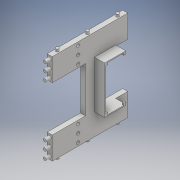
# Autodesk Inventor part: Side Panels V2
Saved by Autodesk Inventor 2017.3 (Build 213256000, 256)
## iProperties
Created: 2018-03-06
Part Number: Side Panels V2
Material: Generic
Document SubType Name: Modeling
Designer: Harsh Gupta
Density: 1 g/cm^3
Appearance: Default
Author: Harsh Gupta
Autodesk Inventor part; units mm, degrees
ref_plane "YZ Plane" through (0, 0, 0) normal (1, 0, 0) x (0, 1, 0)
sketch "Sketch1" plane through (0, 0, 0) normal (0, 1, 0) x (-1, 0, 0)
  line L0 (0, 0) -> (5, 0)
  line L1 (5, 0) -> (5, -90)
  line L2 (5, -90) -> (0, -90)
  line L3 (0, -90) -> (0, 0)
  dimension "d0" = 5
  dimension "d1" = 90
  constraints: 8 end point, 2 parallel, 1 horizontal, 1 perpendicular
  measures "d0" distance of L1.end L2.end
  measures "d1" distance of L0.end L1.end
extrude "Extrusion1" add sketch "Sketch1" along normal blind 75
sketch "Sketch2" plane through (0, 0, 0) normal (1, 0, 0) x (0, 0, -1)
  line L0 (90, 0) -> (0, 0) projected
  line L1 (22.5, 0) -> (67.5, 0)
  line L2 (67.5, 0) -> (67.5, 33)
  line L3 (67.5, 33) -> (22.5, 33)
  line L4 (22.5, 33) -> (22.5, 0)
  line L5 (0, 0) -> (0, 75) projected
  line L6 (90, 0) -> (90, 75) projected
  line L7 (22.5, 43) -> (67.5, 43)
  line L8 (67.5, 43) -> (67.5, 75)
  line L9 (67.5, 75) -> (22.5, 75)
  line L10 (22.5, 75) -> (22.5, 43)
  line L11 (0, 75) -> (90, 75) projected
  dimension "d4" = 45
  dimension "d5" = 22.5
  dimension "d6" = 22.5
  dimension "d7" = 33
  dimension "d8" = 10
  dimension "d9" = 22.5
  dimension "d10" = 22.5
  constraints: 16 end point, 4 parallel, 2 horizontal, 2 perpendicular, 1 collinear, 1 point on line
  measures "d4" distance of L3.end L2.end
  measures "d5" distance between parallel lines of L5 L4
  measures "d6" distance between parallel lines of L6 L2
  measures "d7" distance of L3.end L1.start
  measures "d8" distance between parallel lines of L7 L3
  measures "d9" distance between parallel lines of L5 L10
  measures "d10" distance between parallel lines of L6 L8
extrude "Extrusion2" cut sketch "Sketch2" against normal through all contours L0 L4 L3 L2 | L8 L7 L10 L9
sketch "Sketch3" plane through (0, 0, 0) normal (1, 0, 0) x (0, 0, -1)
  line L0 (67.5, 43) -> (22.5, 43) projected
  line L1 (67.5, 63) -> (67.5, 43) projected
  line L2 (22.5, 63) -> (67.5, 63) projected
  line L3 (22.5, 43) -> (22.5, 63) projected
  circle A0 centre (23.5, 44) radius 0.75 projected
  circle A1 centre (23.5, 62) radius 0.75 projected
  circle A2 centre (66.5, 44) radius 0.75 projected
  circle A3 centre (66.5, 62) radius 0.75 projected
  line L4 (42.55, 45.5) -> (42.35, 45.5) projected
  line L5 (42.55, 45.5) -> (42.65, 45.6) projected
  line L6 (44.8, 45.6) -> (42.65, 45.6) projected
  line L7 (44.8, 45.6) -> (44.9, 45.5) projected
  line L8 (45.1, 45.5) -> (44.9, 45.5) projected
  line L9 (45.1, 45.5) -> (45.2, 45.6) projected
  line L10 (47.35, 45.6) -> (45.2, 45.6) projected
  line L11 (47.35, 45.6) -> (47.45, 45.5) projected
  line L12 (47.65, 45.5) -> (47.45, 45.5) projected
  line L13 (47.65, 45.5) -> (47.75, 45.6) projected
  line L14 (49.9, 45.6) -> (47.75, 45.6) projected
  line L15 (49.9, 45.6) -> (50, 45.5) projected
  line L16 (50, 43.2) -> (50, 45.5) projected
  line L17 (50, 43.2) -> (49.9, 43.1) projected
  line L18 (47.75, 43.1) -> (49.9, 43.1) projected
  line L19 (47.75, 43.1) -> (47.65, 43.2) projected
  line L20 (47.45, 43.2) -> (47.65, 43.2) projected
  line L21 (47.45, 43.2) -> (47.35, 43.1) projected
  line L22 (45.2, 43.1) -> (47.35, 43.1) projected
  line L23 (45.2, 43.1) -> (45.1, 43.2) projected
  line L24 (44.9, 43.2) -> (45.1, 43.2) projected
  line L25 (44.9, 43.2) -> (44.8, 43.1) projected
  line L26 (42.65, 43.1) -> (44.8, 43.1) projected
  line L27 (42.65, 43.1) -> (42.55, 43.2) projected
  line L28 (42.35, 43.2) -> (42.55, 43.2) projected
  line L29 (42.35, 43.2) -> (42.25, 43.1) projected
  line L30 (40.1, 43.1) -> (42.25, 43.1) projected
  line L31 (40.1, 43.1) -> (40, 43.2) projected
  line L32 (40, 45.5) -> (40, 43.2) projected
  line L33 (40, 45.5) -> (40.1, 45.6) projected
  line L34 (42.25, 45.6) -> (40.1, 45.6) projected
  line L35 (42.25, 45.6) -> (42.35, 45.5) projected
  line L36 (24, 56.95) -> (24, 56.75) projected
  line L37 (24.1, 56.95) -> (24, 56.95) projected
  line L38 (24.1, 56.75) -> (24.1, 56.95) projected
  line L39 (24, 56.75) -> (24.1, 56.75) projected
  line L40 (28.9, 56.95) -> (28.9, 56.75) projected
  line L41 (29, 56.95) -> (28.9, 56.95) projected
  line L42 (29, 56.75) -> (29, 56.95) projected
  line L43 (28.9, 56.75) -> (29, 56.75) projected
  line L44 (24, 55.8071) -> (24, 55.6071) projected
  line L45 (24.1, 55.8071) -> (24, 55.8071) projected
  line L46 (24.1, 55.6071) -> (24.1, 55.8071) projected
  line L47 (24, 55.6071) -> (24.1, 55.6071) projected
  line L48 (28.9, 55.8071) -> (28.9, 55.6071) projected
  line L49 (29, 55.8071) -> (28.9, 55.8071) projected
  line L50 (29, 55.6071) -> (29, 55.8071) projected
  line L51 (28.9, 55.6071) -> (29, 55.6071) projected
  line L52 (24, 54.6643) -> (24, 54.4643) projected
  line L53 (24.1, 54.6643) -> (24, 54.6643) projected
  line L54 (24.1, 54.4643) -> (24.1, 54.6643) projected
  line L55 (24, 54.4643) -> (24.1, 54.4643) projected
  line L56 (28.9, 54.6643) -> (28.9, 54.4643) projected
  line L57 (29, 54.6643) -> (28.9, 54.6643) projected
  line L58 (29, 54.4643) -> (29, 54.6643) projected
  line L59 (28.9, 54.4643) -> (29, 54.4643) projected
  line L60 (24, 53.5214) -> (24, 53.3214) projected
  line L61 (24.1, 53.5214) -> (24, 53.5214) projected
  line L62 (24.1, 53.3214) -> (24.1, 53.5214) projected
  line L63 (24, 53.3214) -> (24.1, 53.3214) projected
  line L64 (28.9, 53.5214) -> (28.9, 53.3214) projected
  line L65 (29, 53.5214) -> (28.9, 53.5214) projected
  line L66 (29, 53.3214) -> (29, 53.5214) projected
  line L67 (28.9, 53.3214) -> (29, 53.3214) projected
  line L68 (24, 52.3786) -> (24, 52.1786) projected
  line L69 (24.1, 52.3786) -> (24, 52.3786) projected
  line L70 (24.1, 52.1786) -> (24.1, 52.3786) projected
  line L71 (24, 52.1786) -> (24.1, 52.1786) projected
  line L72 (28.9, 52.3786) -> (28.9, 52.1786) projected
  line L73 (29, 52.3786) -> (28.9, 52.3786) projected
  line L74 (29, 52.1786) -> (29, 52.3786) projected
  line L75 (28.9, 52.1786) -> (29, 52.1786) projected
  line L76 (24, 51.2357) -> (24, 51.0357) projected
  line L77 (24.1, 51.2357) -> (24, 51.2357) projected
  line L78 (24.1, 51.0357) -> (24.1, 51.2357) projected
  line L79 (24, 51.0357) -> (24.1, 51.0357) projected
  line L80 (28.9, 51.2357) -> (28.9, 51.0357) projected
  line L81 (29, 51.2357) -> (28.9, 51.2357) projected
  line L82 (29, 51.0357) -> (29, 51.2357) projected
  line L83 (28.9, 51.0357) -> (29, 51.0357) projected
  line L84 (24, 50.0929) -> (24, 49.8929) projected
  line L85 (24.1, 50.0929) -> (24, 50.0929) projected
  line L86 (24.1, 49.8929) -> (24.1, 50.0929) projected
  line L87 (24, 49.8929) -> (24.1, 49.8929) projected
  line L88 (28.9, 50.0929) -> (28.9, 49.8929) projected
  line L89 (29, 50.0929) -> (28.9, 50.0929) projected
  line L90 (29, 49.8929) -> (29, 50.0929) projected
  line L91 (28.9, 49.8929) -> (29, 49.8929) projected
  line L92 (24, 48.95) -> (24, 48.75) projected
  line L93 (24.1, 48.95) -> (24, 48.95) projected
  line L94 (24.1, 48.75) -> (24.1, 48.95) projected
  line L95 (24, 48.75) -> (24.1, 48.75) projected
  line L96 (28.9, 48.95) -> (28.9, 48.75) projected
  line L97 (29, 48.95) -> (28.9, 48.95) projected
  line L98 (29, 48.75) -> (29, 48.95) projected
  line L99 (28.9, 48.75) -> (29, 48.75) projected
  line L100 (40.95, 50.5) -> (41.15, 50.5) projected
  line L101 (40.95, 50.55) -> (40.95, 50.5) projected
  line L102 (41.15, 50.55) -> (40.95, 50.55) projected
  line L103 (41.15, 50.5) -> (41.15, 50.55) projected
  line L104 (41.15, 55.5) -> (40.95, 55.5) projected
  line L105 (41.15, 55.45) -> (41.15, 55.5) projected
  line L106 (40.95, 55.45) -> (41.15, 55.45) projected
  line L107 (40.95, 55.5) -> (40.95, 55.45) projected
  line L108 (42.2667, 50.5) -> (42.4667, 50.5) projected
  line L109 (42.2667, 50.55) -> (42.2667, 50.5) projected
  line L110 (42.4667, 50.55) -> (42.2667, 50.55) projected
  line L111 (42.4667, 50.5) -> (42.4667, 50.55) projected
  line L112 (42.4667, 55.5) -> (42.2667, 55.5) projected
  line L113 (42.4667, 55.45) -> (42.4667, 55.5) projected
  line L114 (42.2667, 55.45) -> (42.4667, 55.45) projected
  line L115 (42.2667, 55.5) -> (42.2667, 55.45) projected
  line L116 (43.5833, 50.5) -> (43.7833, 50.5) projected
  line L117 (43.5833, 50.55) -> (43.5833, 50.5) projected
  line L118 (43.7833, 50.55) -> (43.5833, 50.55) projected
  line L119 (43.7833, 50.5) -> (43.7833, 50.55) projected
  line L120 (43.7833, 55.5) -> (43.5833, 55.5) projected
  line L121 (43.7833, 55.45) -> (43.7833, 55.5) projected
  line L122 (43.5833, 55.45) -> (43.7833, 55.45) projected
  line L123 (43.5833, 55.5) -> (43.5833, 55.45) projected
  line L124 (44.9, 50.5) -> (45.1, 50.5) projected
  line L125 (44.9, 50.55) -> (44.9, 50.5) projected
  line L126 (45.1, 50.55) -> (44.9, 50.55) projected
  line L127 (45.1, 50.5) -> (45.1, 50.55) projected
  line L128 (45.1, 55.5) -> (44.9, 55.5) projected
  line L129 (45.1, 55.45) -> (45.1, 55.5) projected
  line L130 (44.9, 55.45) -> (45.1, 55.45) projected
  line L131 (44.9, 55.5) -> (44.9, 55.45) projected
  line L132 (46.2167, 50.5) -> (46.4167, 50.5) projected
  line L133 (46.2167, 50.55) -> (46.2167, 50.5) projected
  line L134 (46.4167, 50.55) -> (46.2167, 50.55) projected
  line L135 (46.4167, 50.5) -> (46.4167, 50.55) projected
  line L136 (46.4167, 55.5) -> (46.2167, 55.5) projected
  line L137 (46.4167, 55.45) -> (46.4167, 55.5) projected
  line L138 (46.2167, 55.45) -> (46.4167, 55.45) projected
  line L139 (46.2167, 55.5) -> (46.2167, 55.45) projected
  line L140 (47.5333, 50.5) -> (47.7333, 50.5) projected
  line L141 (47.5333, 50.55) -> (47.5333, 50.5) projected
  line L142 (47.7333, 50.55) -> (47.5333, 50.55) projected
  line L143 (47.7333, 50.5) -> (47.7333, 50.55) projected
  line L144 (47.7333, 55.5) -> (47.5333, 55.5) projected
  line L145 (47.7333, 55.45) -> (47.7333, 55.5) projected
  line L146 (47.5333, 55.45) -> (47.7333, 55.45) projected
  line L147 (47.5333, 55.5) -> (47.5333, 55.45) projected
  line L148 (48.85, 50.5) -> (49.05, 50.5) projected
  line L149 (48.85, 50.55) -> (48.85, 50.5) projected
  line L150 (49.05, 50.55) -> (48.85, 50.55) projected
  line L151 (49.05, 50.5) -> (49.05, 50.55) projected
  line L152 (49.05, 55.5) -> (48.85, 55.5) projected
  line L153 (49.05, 55.45) -> (49.05, 55.5) projected
  line L154 (48.85, 55.45) -> (49.05, 55.45) projected
  line L155 (48.85, 55.5) -> (48.85, 55.45) projected
  line L156 (59.1, 50.5) -> (59.3, 50.5) projected
  line L157 (59.1, 50.55) -> (59.1, 50.5) projected
  line L158 (59.3, 50.55) -> (59.1, 50.55) projected
  line L159 (59.3, 50.5) -> (59.3, 50.55) projected
  line L160 (59.3, 55.5) -> (59.1, 55.5) projected
  line L161 (59.3, 55.45) -> (59.3, 55.5) projected
  line L162 (59.1, 55.45) -> (59.3, 55.45) projected
  line L163 (59.1, 55.5) -> (59.1, 55.45) projected
  line L164 (60.4167, 50.5) -> (60.6167, 50.5) projected
  line L165 (60.4167, 50.55) -> (60.4167, 50.5) projected
  line L166 (60.6167, 50.55) -> (60.4167, 50.55) projected
  line L167 (60.6167, 50.5) -> (60.6167, 50.55) projected
  line L168 (60.6167, 55.5) -> (60.4167, 55.5) projected
  line L169 (60.6167, 55.45) -> (60.6167, 55.5) projected
  line L170 (60.4167, 55.45) -> (60.6167, 55.45) projected
  line L171 (60.4167, 55.5) -> (60.4167, 55.45) projected
  line L172 (61.7333, 50.5) -> (61.9333, 50.5) projected
  line L173 (61.7333, 50.55) -> (61.7333, 50.5) projected
  line L174 (61.9333, 50.55) -> (61.7333, 50.55) projected
  line L175 (61.9333, 50.5) -> (61.9333, 50.55) projected
  line L176 (61.9333, 55.5) -> (61.7333, 55.5) projected
  line L177 (61.9333, 55.45) -> (61.9333, 55.5) projected
  line L178 (61.7333, 55.45) -> (61.9333, 55.45) projected
  line L179 (61.7333, 55.5) -> (61.7333, 55.45) projected
  line L180 (63.05, 50.5) -> (63.25, 50.5) projected
  line L181 (63.05, 50.55) -> (63.05, 50.5) projected
  line L182 (63.25, 50.55) -> (63.05, 50.55) projected
  line L183 (63.25, 50.5) -> (63.25, 50.55) projected
  line L184 (63.25, 55.5) -> (63.05, 55.5) projected
  line L185 (63.25, 55.45) -> (63.25, 55.5) projected
  line L186 (63.05, 55.45) -> (63.25, 55.45) projected
  line L187 (63.05, 55.5) -> (63.05, 55.45) projected
  line L188 (64.3667, 50.5) -> (64.5667, 50.5) projected
  line L189 (64.3667, 50.55) -> (64.3667, 50.5) projected
  line L190 (64.5667, 50.55) -> (64.3667, 50.55) projected
  line L191 (64.5667, 50.5) -> (64.5667, 50.55) projected
  line L192 (64.5667, 55.5) -> (64.3667, 55.5) projected
  line L193 (64.5667, 55.45) -> (64.5667, 55.5) projected
  line L194 (64.3667, 55.45) -> (64.5667, 55.45) projected
  line L195 (64.3667, 55.5) -> (64.3667, 55.45) projected
  line L196 (65.6833, 50.5) -> (65.8833, 50.5) projected
  line L197 (65.6833, 50.55) -> (65.6833, 50.5) projected
  line L198 (65.8833, 50.55) -> (65.6833, 50.55) projected
  line L199 (65.8833, 50.5) -> (65.8833, 50.55) projected
  line L200 (65.8833, 55.5) -> (65.6833, 55.5) projected
  line L201 (65.8833, 55.45) -> (65.8833, 55.5) projected
  line L202 (65.6833, 55.45) -> (65.8833, 55.45) projected
  line L203 (65.6833, 55.5) -> (65.6833, 55.45) projected
  line L204 (67, 50.5) -> (67.2, 50.5) projected
  line L205 (67, 50.55) -> (67, 50.5) projected
  line L206 (67.2, 50.55) -> (67, 50.55) projected
  line L207 (67.2, 50.5) -> (67.2, 50.55) projected
  line L208 (67.2, 55.5) -> (67, 55.5) projected
  line L209 (67.2, 55.45) -> (67.2, 55.5) projected
  line L210 (67, 55.45) -> (67.2, 55.45) projected
  line L211 (67, 55.5) -> (67, 55.45) projected
  line L212 (58.9, 55) -> (58.9, 51) projected
  line L213 (67.4, 55) -> (58.9, 55) projected
  line L214 (67.4, 51) -> (67.4, 55) projected
  line L215 (58.9, 51) -> (67.4, 51) projected
  line L216 (49.25, 51) -> (49.25, 55) projected
  line L217 (40.75, 51) -> (49.25, 51) projected
  line L218 (40.75, 55) -> (40.75, 51) projected
  line L219 (49.25, 55) -> (40.75, 55) projected
  line L220 (24.5, 57.75) -> (24.5, 48.25) projected
  line L221 (28.5, 57.75) -> (24.5, 57.75) projected
  line L222 (28.5, 48.25) -> (28.5, 57.75) projected
  line L223 (24.5, 48.25) -> (28.5, 48.25) projected
  line L224 (22.5, 63) -> (21.5, 63)
  line L225 (21.5, 63) -> (21.5, 42)
  line L226 (21.5, 42) -> (22.5, 42)
  line L227 (22.5, 43) -> (22.5, 63)
  line L228 (67.5, 63) -> (68.5, 63)
  line L229 (68.5, 63) -> (68.5, 42)
  line L230 (68.5, 42) -> (67.5, 42)
  line L231 (67.5, 43) -> (67.5, 63)
  line L232 (67.5, 75) -> (67.5, 43) projected
  line L233 (22.5, 42) -> (67.5, 42)
  line L234 (67.5, 43) -> (22.5, 43)
  point P0 (0, 0)
  dimension "d13" = 1
  dimension "d14" = 21
  dimension "d15" = 1
  dimension "d17" = 47
  constraints: 20 end point, 5 parallel, 3 horizontal, 2 perpendicular, 2 point on line, 1 collinear
  measures "d13" distance of L226.end L225.end
  measures "d14" distance of L225.end L224.end
  measures "d15" distance of L229.end L230.end
  measures "d17" distance of L225.end L229.end
extrude "Extrusion3" add sketch "Sketch3" along normal blind 10 contours L1 L228 L229 L230 L233 L226 L225 L224 L3 L0
ref_plane "Work Plane1" through (8.43, 53, 385.6573) normal (1, 0, 0) x (0, 0, -1)
sketch "Sketch4" plane through (8.43, 53, 385.6573) normal (1, 0, 0) x (0, 0, -1)
  line L0 (408.1573, -10) -> (408.1573, 10) projected
  line L1 (408.1573, 10) -> (410.1573, 10)
  line L2 (410.1573, 10) -> (410.1573, 8)
  line L3 (410.1573, 8) -> (408.1573, 8)
  line L4 (408.1573, 8) -> (408.1573, 10)
  line L5 (453.1573, -10) -> (408.1573, -10) projected
  line L6 (408.1573, -10) -> (410.1573, -10)
  line L7 (410.1573, -10) -> (410.1573, -8)
  line L8 (410.1573, -8) -> (408.1573, -8)
  line L9 (408.1573, -8) -> (408.1573, -10)
  line L10 (234.5466, 10) -> (234.5466, -10) projected
  line L11 (453.1573, -10) -> (451.1573, -10)
  line L12 (451.1573, -10) -> (451.1573, -8)
  line L13 (451.1573, -8) -> (453.1573, -8)
  line L14 (453.1573, -8) -> (453.1573, -10)
  line L15 (453.1573, 10) -> (451.1573, 10)
  line L16 (451.1573, 10) -> (451.1573, 8)
  line L17 (451.1573, 8) -> (453.1573, 8)
  line L18 (453.1573, 8) -> (453.1573, 10)
  point P0 (385.6573, -53)
  dimension "d20" = 2
  dimension "d21" = 2
  dimension "d22" = 2
  dimension "d23" = 2
  dimension "d24" = 2
  dimension "d25" = 2
  dimension "d26" = 2
  dimension "d27" = 2
  constraints: 32 end point, 8 parallel, 4 horizontal, 4 perpendicular
  measures "d20" distance of L2.end L3.end
  measures "d21" distance of L1.end L2.end
  measures "d22" distance of L8.end L7.end
  measures "d23" distance of L7.end L6.end
  measures "d24" distance of L12.end L13.end
  measures "d25" distance of L11.end L12.end
  measures "d26" distance of L17.end L16.end
  measures "d27" distance of L16.end L15.end
extrude "Extrusion4" add sketch "Sketch4" along normal up to surface (1.57 mm away)
sketch "Sketch5" plane through (0, 0, 0) normal (0, -1, 0) x (1, 0, 0)
  circle A0 centre (-2.5, -3.25) radius 1.5
  line L0 (-5, 0) -> (-5, -22.5) projected
  line L1 (0, 0) -> (-5, 0) projected
  line L2 (-5, -22.5) -> (0, -22.5) projected
  dimension "d30" = 3
  dimension "d31" = 2.5
  dimension "d32" = 3.25
  constraints: 1 centre point
  measures "d30" diameter of A0
  measures "d31" distance from line of L0 A0.centre
  measures "d32" distance from line of L1 A0.centre
extrude "Extrusion5" add sketch "Sketch5" along normal blind 5
pattern_linear "Rectangular Pattern1" count 3 spacing 8 along (0, 0, -1) of "Extrusion5"
sketch "Sketch7" plane through (0, 0, 0) normal (0, -1, 0) x (1, 0, 0)
  circle A0 centre (-2.5, -86.75) radius 1.5
  line L0 (-5, -67.5) -> (-5, -90) projected
  line L1 (-5, -90) -> (0, -90) projected
  point P0 (0, 0)
  dimension "d40" = 3
  dimension "d41" = 2.5
  dimension "d42" = 3.25
  constraints: 1 centre point
  measures "d40" diameter of A0
  measures "d41" distance from line of L0 A0.centre
  measures "d42" distance from line of L1 A0.centre
extrude "Extrusion6" add sketch "Sketch7" along normal blind 5
pattern_linear "Rectangular Pattern2" count 3 spacing 8 along (0, 0, 1) of "Extrusion6"
sketch "Sketch8" plane through (0, 0, 0) normal (1, 0, 0) x (0, 0, -1)
  line L0 (90, 0) -> (90, 75) projected
  line L1 (0, 0) -> (0, 75) projected
  line L2 (90, 23) -> (0, 23)
  line L3 (0, 23) -> (0, 28)
  line L4 (0, 28) -> (90, 28)
  line L5 (90, 28) -> (90, 23)
  line L6 (22.5, 0) -> (0, 0) projected
  circle A0 centre (3.25, 25.5) radius 1.5
  dimension "d48" = 5
  dimension "d49" = 23
  dimension "d50" = 3
  dimension "d51" = 2.5
  dimension "d52" = 3.25
  constraints: 8 end point, 2 parallel, 2 point on line, 1 centre point, 1 horizontal, 1 perpendicular
  measures "d48" distance of L2.end L3.end
  measures "d49" distance between parallel lines of L6 L2
  measures "d50" diameter of A0
  measures "d51" distance from line of L2 A0.centre
  measures "d52" distance from line of L1 A0.centre
extrude "Extrusion7" cut sketch "Sketch8" against normal blind 2.5 contours A0
ref_plane "Work Plane2" through (-5, 0, -45) normal (0, 0, 1) x (1, 0, 0)
pattern_linear "Rectangular Pattern3" count 3 spacing 8 along (0, 0, -1) of "Extrusion7"
mirror "Mirror1" about plane through (-5, 0, -45) normal (0, 0, 1) of "Extrusion7", "Rectangular Pattern3"
sketch "Sketch9" plane through (-5, 0, 0) normal (0, 0, 1) x (1, 0, 0)
  circle A0 centre (2.5, 67.5) radius 1.5
  line L0 (5, 0) -> (5, 75) projected
  line L1 (0, 75) -> (5, 75) projected
  dimension "d59" = 3
  dimension "d60" = 2.5
  dimension "d61" = 7.5
  constraints: 1 centre point
  measures "d59" diameter of A0
  measures "d60" distance from line of L0 A0.centre
  measures "d61" distance from line of L1 A0.centre
extrude "Extrusion8" add sketch "Sketch9" along normal blind 2.5
pattern_linear "Rectangular Pattern4" count 3 spacing 30 along (0, -1, 0) of "Extrusion8"
mirror "Mirror2" about plane through (-5, 0, -45) normal (0, 0, 1) of "Extrusion8", "Rectangular Pattern4"
equation "\"d5\" = d6"
equation "\"d10\" = d9"
body "Solid1"
